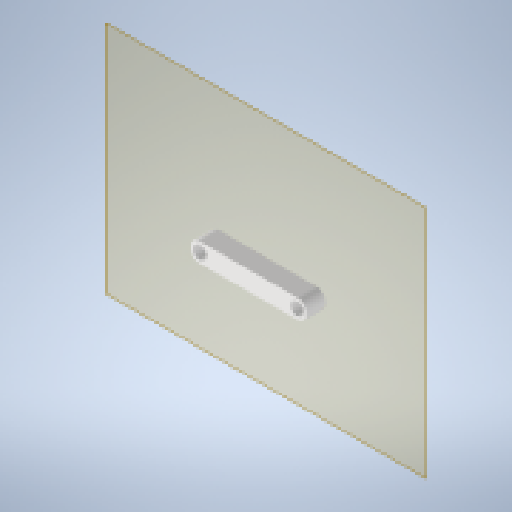
# Autodesk Inventor part: TinyBeltClamp
Saved by Autodesk Inventor 2023 (Build 270158000, 158)
## iProperties
Created: 2023-09-08
Part Number: TinyBeltClamp
Material: Generic
Document SubType Name: Modeling
Designer: Felix
Density: 1 g/cm^3
Appearance: Default
Author: Felix
Autodesk Inventor part; units mm, degrees
ref_plane "YZ Plane" through (0, 0, 0) normal (1, 0, 0) x (0, 1, 0)
ref_plane "XZ Plane" through (0, 0, 0) normal (0, 1, 0) x (-1, 0, 0)
ref_plane "XY Plane" through (0, 0, 0) normal (0, 0, 1) x (1, 0, 0)
ref_plane "Work Plane1" through (0, 0, 0) normal (0, 0, 1) x (1, 0, 0)
sketch "Sketch1" plane through (0, 0, 0) normal (0, 0, 1) x (1, 0, 0)
  circle A0 centre (-12.1, 23.75) radius 2.15 construction
  circle A1 centre (13.2, 23.75) radius 2.15 construction
  circle A2 centre (-12.1, 31.75) radius 2.15 construction
  circle A3 centre (13.2, 31.75) radius 2.15 construction
  line L0 (-12.1, 23.75) -> (13.2, 23.75) construction
  line L1 (-12.1, 21.25) -> (13.2, 21.25)
  line L2 (13.2, 26.25) -> (-12.1, 26.25)
  arc A4 (-12.1, 26.25) -> (-12.1, 21.25) centre (-12.1, 23.75) ccw
  arc A5 (13.2, 21.25) -> (13.2, 26.25) centre (13.2, 23.75) ccw
  point P0 (0, 0)
  point P1 (0.55, 23.75)
  dimension "d0" = 5
  constraints: 8 end point, 4 point on circle, 4 tangent, 2 centre point, 1 horizontal, 1 midpoint, 1 parallel
  measures "d0" diameter of A5
extrude "Extrusion1" add sketch "Sketch1" along normal blind 5
sketch "Sketch2" plane through (0, 0, 5) normal (0, 0, 1) x (1, 0, 0)
  arc A0 (13.2, 21.25) -> (13.2, 26.25) centre (13.2, 23.75) ccw construction
  line L0 (13.2, 26.25) -> (-12.1, 26.25) construction
  arc A1 (-12.1, 26.25) -> (-12.1, 21.25) centre (-12.1, 23.75) ccw construction
  line L1 (-12.1, 21.25) -> (13.2, 21.25) construction
  point P0 (0, 0)
  constraints: 2 coincident
hole "Hole1" at (13.2, 23.75, 5) at (-12.1, 23.75, 5) direction (0, 0, -1) diameter 3.4 depth 7 clearance for "Countersunk Flat Head Screw DIN EN ISO 2009" size "M3" standard "DIN"
body "Solid1"
